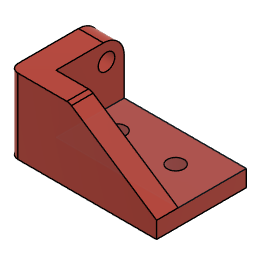
GTMS TEMPLATE (Autodesk Fusion 360 archive; units mm, degrees)
design "ROOF MOUNT"
Autodesk Fusion 360 part; units mm, degrees
(part 1 of 24)
sketch "Sketch1" plane through (0, 0, 0) normal (0, 1, 0) x (1, 0, 0)
sketch "Sketch2" plane through (0, 0, 0) normal (0, 0, 1) x (1, 0, 0)
  line L0 (0, 0) -> (7.2, 0)
  line L1 (7.2, 0) -> (7.2, 3)
  line L2 (7.2, 3) -> (14.4, 3)
  line L3 (14.4, 3) -> (14.4, 0)
  line L4 (14.4, 0) -> (17.7, 0)
  line L5 (17.7, 0) -> (17.7, 3)
  line L6 (0, 0) -> (0, 10)
  line L7 (0, 10) -> (7.2, 10)
  line L8 (7.2, 10) -> (17.7, 3)
  dimension "d1" = 7.2
  dimension "d2" = 3
  dimension "d3" = 7.2
  dimension "d4" = 3.3
  dimension "d5" = 3
  dimension "d6" = 10
  dimension "d7" = 7.2
  constraint coincident L0.start L6.start
  constraint horizontal L0
  constraint perpendicular L0 L1
  constraint perpendicular L1 L2
  constraint perpendicular L2 L3
  constraint perpendicular L3 L4
  constraint perpendicular L4 L5
  constraint perpendicular L0 L6
  constraint perpendicular L6 L7
  measures "d1" distance of L0.start L0.end
  measures "d2" distance of L0.end L1.end
  measures "d3" distance of L1.end L2.end
  measures "d4" distance of L3.end L4.end
  measures "d5" distance of L4.end L5.end
  measures "d6" distance of L0.start L6.end
  measures "d7" distance of L6.end L7.end
ref_plane "WorkPlane1" through (0, 0, 0) normal (1, 0, 0) x (0, 1, 0)
sketch "Sketch3" plane through (0, 0, 0) normal (1, 0, 0) x (0, 0, -1)
extrude "Extrude1" add sketch "Sketch2" against normal blind 2.6
sketch "Sketch4" plane through (0, 0, 0) normal (1, 0, 0) x (0, 0, -1)
  line L0 (2.6, 0) -> (10.8, 0)
  line L1 (10.8, 0) -> (10.8, 3)
  line L2 (10.8, 3) -> (2.6, 3)
  line L3 (2.6, 3) -> (2.6, 0)
  line L4 (2.6, 10) -> (8.8, 10)
  line L5 (10.8, 8) -> (10.8, 3)
  line L6 (10.8, 3) -> (2.6, 3)
  line L7 (2.6, 3) -> (2.6, 10)
  circle A0 centre (8.6724, 7.8369) radius 1
  line L8 (8.8, 10) -> (10.8, 10)
  line L9 (10.8, 10) -> (10.8, 8)
  point P0 (10.8, 10)
  dimension "d11" = 8.2
  dimension "d12" = 3
  dimension "d13" = 8.2
  dimension "d14" = 3
  dimension "d16" = 8.2
  dimension "d18" = 2
  constraint horizontal L0
  constraint perpendicular L0 L1
  constraint perpendicular L1 L2
  constraint perpendicular L2 L3
  constraint horizontal L4
  constraint perpendicular L2 L5
  constraint coincident P0 L4
  constraint coincident P0 L5
  constraint coincident P0 L8.end
  measures "d11" distance of L0.start L0.end
  measures "d12" distance of L0.end L1.end
  measures "d13" distance of L1.end L2.end
  measures "d14" distance of L2.end L0.start
  measures "d16" distance of L4.start P0
  measures "d18" diameter of A0
extrude "Extrude2" add sketch "Sketch4" along normal blind 3 contours L2 L4 L5 L6 L7 L8 L9
extrude "Extrude3" add sketch "Sketch4" along normal blind 7.2 contours L0 L1 L2 L3 L6
fillet "Fillet2" radius 1 1 edges at (7.2, 10, -1.3)
fillet "Fillet3" radius 1 1 edges at (0, 5, 0)
fillet "Fillet5" radius 1 1 edges at (16.05, 0, 0)
sketch "Sketch5" plane through (0, 0, 0) normal (0, 0, 1) x (1, 0, 0)
extrude "Extrude4" add sketch "Sketch4" along normal blind 3 contours L2 L4 L5 L6 L7 L8 L9
fillet "Fillet6" radius 2.5 1 edges at (1.5, 10, -10.8)
extrude "Extrude5" cut 1 faces at (7.2, 1, -4.4667) along direction (1, 0, 0) blind 12
extrude "Extrude6" add 1 faces at (7.2, 1, -4.4667) along direction (1, 0, 0) blind 10.5
extrude "Extrude7" cut 1 faces at (6.2333, 0, -7.2) along direction (0, 1, 0) blind 1
sketch "Sketch6" plane through (0, 3, 0) normal (0, 1, 0) x (-1, 0, 0)
  line L0 (-3, -10.8) -> (-3, -2.6)
  line L1 (-3, -2.6) -> (-17.7, -2.6)
  line L2 (-17.7, -2.6) -> (-17.7, -10.8)
  line L3 (-17.7, -10.8) -> (-3, -10.8)
sketch "Sketch7" plane through (0, 3, 0) normal (0, 1, 0) x (-1, 0, 0)
  circle A0 centre (-6, -7) radius 1
  circle A1 centre (-13, -7) radius 1
  dimension "d43" = 2
  dimension "d44" = 2
  measures "d43" diameter of A0
  measures "d44" diameter of A1
hole "Hole1" at (6, 3, -7) direction (0, -1, 0) diameter 2 depth 4 tip angle 118
hole "Hole2" at (13, 3, -7) direction (0, -1, 0) diameter 2 depth 4 tip angle 118

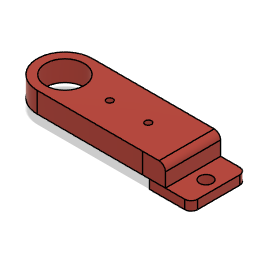
design "SERVO CAM"
Autodesk Fusion 360 part; units mm, degrees
sketch "Sketch1" plane through (0, 0, 0) normal (0, 1, 0) x (1, 0, 0)
  circle A0 centre (0, 0) radius 2.5
  line L0 (-0.0213, 4.2999) -> (16.4103, 4.3)
  line L1 (-0.0213, -4.2999) -> (16.4103, -4.3)
  arc A1 (0.0212, 4.2999) -> (0.0212, -4.2999) centre (0, 0) ccw
  arc A2 (16.3897, -4.3) -> (16.3897, 4.3) centre (16.4, 0) ccw
  point P0 (-4.3, 0)
  point P1 (25.7, 0)
  dimension "d1" = 5
  dimension "d2" = 8.6
  dimension "d12" = 16.4
  dimension "d14" = 8.6
  constraint coincident A0.centre A1.centre
  constraint concentric A0 A1
  constraint coincident L0.start A1
  constraint coincident L1.start A1
  constraint coincident L0 A1.start
  constraint coincident L1 A1.end
  constraint midpoint A1 P0
  constraint coincident L0.end A2
  constraint coincident L1.end A2
  constraint coincident L0 A2.end
  constraint coincident L1 A2.start
  measures "d1" diameter of A0
  measures "d2" diameter of A1
  measures "d12" distance of A0.centre A2.centre
  measures "d14" diameter of A2
sketch "Sketch2" plane through (0, 0, 0) normal (0, 1, 0) x (1, 0, 0)
  point P0 (-0.8314, -7.8419)
sketch "Sketch3" plane through (0, 0, 0) normal (0, 1, 0) x (1, 0, 0)
  circle A0 centre (18.5, 0) radius 1
  dimension "d16" = 2
  measures "d16" diameter of A0
extrude "Extrude2" add sketch "Sketch1" along normal blind 3.2
extrude "Extrude3" cut sketch "Sketch3" along normal blind 12
sketch "Sketch4" plane through (0, 3.2, 0) normal (0, 1, 0) x (-1, 0, 0)
  circle A0 centre (-18.5, 0) radius 1
  circle A1 centre (0, 0) radius 2.5
  arc A2 (0.0213, -4.2999) -> (0.0213, 4.2999) centre (0, 0) ccw
  line L0 (0.0213, 4.2999) -> (-16.4103, 4.3)
  arc A3 (-16.4103, 4.3) -> (-16.4103, -4.3) centre (-16.4, 0) ccw
  line L1 (-16.4103, -4.3) -> (0.0213, -4.2999)
  line L2 (-16.4103, 4.3) -> (-16.4103, -4.3)
  constraint coincident L0.end A3.start
  constraint coincident A3.end L1.start
extrude "Extrude4" cut sketch "Sketch4" against normal blind 3 contours A3 L2
extrude "Extrude5" cut 1 faces at (16.7735, 0.2, 0) along direction (0, -1, 0) blind 0.5
sketch "Sketch5" plane through (0, 0, 0) normal (0, 1, 0) x (1, 0, 0)
sketch "Sketch6" plane through (16.4103, 0, 0) normal (1, 0, 0) x (0, 0, -1)
  line L0 (4.3, 3.2) -> (-4.3, 3.2)
  line L1 (-4.3, 3.2) -> (-4.3, 0)
  line L2 (-4.3, 0) -> (4.3, 0)
  line L3 (4.3, 0) -> (4.3, 3.2)
sketch "Sketch7" plane through (0, 0, 0) normal (0, 1, 0) x (1, 0, 0)
extrude "Extrude6" add sketch "Sketch6" along normal blind 3.568
sketch "Sketch8" plane through (0, 0, 0) normal (0, 1, 0) x (1, 0, 0)
  line L0 (19.98, -4.3) -> (16.98, -4.3)
  line L1 (19.98, -4.3) -> (23.98, -4.3)
  line L2 (23.98, -4.3) -> (23.98, 7.4552)
  line L3 (20, 4.3) -> (23.98, 4.3)
  line L4 (20, 4.3) -> (17, 4.3)
  line L5 (16.98, -4.3) -> (17, 4.3)
  dimension "d33" = 3
  dimension "d34" = 4
  dimension "d35" = 3
  constraint horizontal L0
  constraint parallel L0 L1
  constraint perpendicular L1 L2
  constraint coincident L2 L3.end
  constraint perpendicular L2 L3
  constraint perpendicular L2 L4
  measures "d33" distance of L0.start L0.end
  measures "d34" distance of L0.start L1.end
  measures "d35" distance of L3.start L4.end
extrude "Extrude7" add sketch "Sketch8" against normal blind 1.4
fillet "Fillet1" radius 1 1 edges at (19.9783, 3.2, 0)
fillet "Fillet2" radius 1 1 edges at (23.98, -0.7, 4.3)
fillet "Fillet3" radius 1 1 edges at (23.98, -0.7, -4.3)
hole "Hole1" at (0, 3.2, 0) direction (0, -1, 0) diameter 6 depth 6 tip angle 180
sketch "Sketch9" plane through (0, 0, 0) normal (0, 1, 0) x (1, 0, 0)
  line L0 (0, 0) -> (26, 0)
  line L1 (20, 3) -> (24, 3)
  line L2 (24, 3) -> (22, 3)
  line L3 (22, 3) -> (22, -3)
  circle A0 centre (22, 0) radius 1
  dimension "d47" = 2
  dimension "d48" = 2
  constraint coincident L0.start origin
  constraint horizontal L0
  constraint parallel L0 L1
  constraint midpoint L1 L2.end
  constraint perpendicular L0 L3
  constraint midpoint L3 A0.centre
  measures "d47" distance of L1.end L2.end
  measures "d48" diameter of A0
hole "Hole2" at (22, 0, 0) direction (0, -1, 0) diameter 2 depth 6 tip angle 180
extrude "Extrude8" cut 1 faces at (16.9867, -0.9333, 1.4333) along direction (0.999997, 0, 0.002325) blind 0.5
delete_face "DeleteFace1" 1 faces at (17.1684, -0.9333, -4.2996)
sketch "Sketch10" plane through (0, 3.2, 0) normal (0, 1, 0) x (-1, 0, 0)
  circle A0 centre (0, 0) radius 3
  line L0 (-18.9783, 4.3) -> (-18.9783, -4.3)
  line L1 (-18.9783, -4.3) -> (-16.4103, -4.3)
  line L2 (-16.4103, -4.3) -> (0.0213, -4.2999)
  arc A1 (0.0213, -4.2999) -> (0.0213, 4.2999) centre (0, 0) ccw
  line L3 (0.0213, 4.2999) -> (-16.4103, 4.3)
  line L4 (-16.4103, 4.3) -> (-18.9783, 4.3)
  line L5 (-3, 0) -> (-4.5, 0)
  line L6 (-4.5, 0) -> (-5, 0)
  circle A2 centre (-5, 0) radius 0.5
  line L7 (-5.5, 0) -> (-6.5, 0)
  line L8 (-6.5, 0) -> (-7, 0)
  circle A3 centre (-7, 0) radius 0.5
  line L9 (-7.5, 0) -> (-8.5, 0)
  line L10 (-8.5, 0) -> (-9, 0)
  circle A4 centre (-9, 0) radius 0.5
  line L11 (-9.5, 0) -> (-10.5, 0)
  line L12 (-10.5, 0) -> (-11, 0)
  circle A5 centre (-11, 0) radius 0.5
  line L13 (-11.5, 0) -> (-12.5, 0)
  line L14 (-12.5, 0) -> (-13, 0)
  circle A6 centre (-13, 0) radius 0.5
  line L15 (-13.5, 0) -> (-14.5, 0)
  line L16 (-14.5, 0) -> (-15, 0)
  circle A7 centre (-15, 0) radius 0.5
  dimension "d54" = 1.5
  dimension "d55" = 0.5
  dimension "d56" = 1
  dimension "d57" = 1
  dimension "d58" = 0.5
  dimension "d59" = 1
  dimension "d60" = 1
  dimension "d61" = 0.5
  dimension "d62" = 1
  dimension "d63" = 1
  dimension "d64" = 0.5
  dimension "d65" = 1
  dimension "d66" = 1
  dimension "d67" = 0.5
  dimension "d68" = 1
  dimension "d69" = 1
  dimension "d70" = 0.5
  dimension "d71" = 1
  constraint coincident A0 L5.start
  constraint horizontal L5
  constraint parallel L2 L6
  constraint coincident L6.end A2.centre
  constraint coincident A2 L7.start
  constraint horizontal L7
  constraint parallel L7 L8
  constraint coincident L8.end A3.centre
  constraint coincident A3 L9.start
  constraint horizontal L9
  constraint parallel L9 L10
  constraint coincident L10.end A4.centre
  constraint coincident A4 L11.start
  constraint horizontal L11
  constraint parallel L11 L12
  constraint coincident L12.end A5.centre
  constraint coincident A5 L13.start
  constraint parallel L2 L13
  constraint horizontal L14
  constraint coincident L14.end A6.centre
  constraint coincident A6 L15.start
  constraint parallel L2 L15
  constraint parallel L15 L16
  constraint coincident L16.end A7.centre
  measures "d54" distance of L5.start L5.end
  measures "d55" distance of L5.end L6.end
  measures "d56" diameter of A2
  measures "d57" distance of L7.start L7.end
  measures "d58" distance of L7.end L8.end
  measures "d59" diameter of A3
  measures "d60" distance of L9.start L9.end
  measures "d61" distance of L9.end L10.end
  measures "d62" diameter of A4
  measures "d63" distance of L11.start L11.end
  measures "d64" distance of L11.end L12.end
  measures "d65" diameter of A5
  measures "d66" distance of L13.start L13.end
  measures "d67" distance of L13.end L14.end
  measures "d68" diameter of A6
  measures "d69" distance of L15.start L15.end
  measures "d70" distance of L15.end L16.end
  measures "d71" diameter of A7
hole "Hole3" at (7, 3.2, 0) direction (0, -1, 0) diameter 1 depth 10 tip angle 118
hole "Hole4" at (13, 3.2, 0) direction (0, -1, 0) diameter 1 depth 10 tip angle 118
extrude "Extrude1" [suppressed]

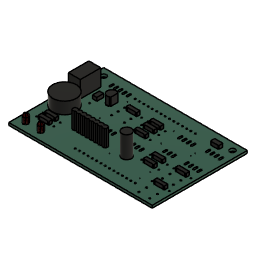
design "IO Daughter Board"
Autodesk Fusion 360 part; units mm, degrees
sketch "Outline" plane through (0, 0, 0) normal (0, 0, 1) x (1, 0, 0)
  line L0 (0, 0) -> (0, 56.3)
  arc A0 (0, 56.3381) -> (0, 56.2619) centre (0, 56.3) ccw
  line L1 (85, 56.3) -> (85, 0)
  arc A1 (85.0381, 56.3) -> (84.9619, 56.3) centre (85, 56.3) ccw
  arc A2 (0.0381, 56.3) -> (-0.0381, 56.3) centre (0, 56.3) ccw
  arc A3 (-0.0381, 0) -> (0.0381, 0) centre (0, 0) ccw
  line L2 (0, 56.3) -> (85, 56.3)
  arc A4 (0, 0.0381) -> (0, -0.0381) centre (0, 0) ccw
  arc A5 (85, 56.2619) -> (85, 56.3381) centre (85, 56.3) ccw
  arc A6 (85, -0.0381) -> (85, 0.0381) centre (85, 0) ccw
  line L3 (85, 0) -> (0, 0)
  arc A7 (84.9619, 0) -> (85.0381, 0) centre (85, 0) ccw
sketch "Top SIlkscreen" plane through (0, 0, 0) normal (0, 0, 1) x (1, 0, 0)
  line L0 (55.2958, 9.3303) -> (56.4642, 9.7197)
  arc A0 (55.2878, 9.3544) -> (55.3038, 9.3062) centre (55.2958, 9.3303) ccw
  arc A1 (52.7304, 13.311) -> (52.7812, 13.311) centre (52.7558, 13.311) ccw
  line L1 (56.1721, 9.6224) -> (56.1721, 9.0382)
  arc A2 (56.4722, 9.6956) -> (56.4562, 9.7438) centre (56.4642, 9.7197) ccw
  arc A3 (53.6646, 12.8425) -> (53.6646, 12.7917) centre (53.6646, 12.8171) ccw
  arc A4 (53.9242, 13.2856) -> (53.9242, 13.3364) centre (53.9242, 13.311) ccw
  arc A5 (53.9242, 10.5777) -> (53.9242, 10.6285) centre (53.9242, 10.6031) ccw
  arc A6 (53.6392, 10.1487) -> (53.69, 10.1487) centre (53.6646, 10.1487) ccw
  arc A7 (52.6347, 11.7855) -> (52.6173, 11.7377) centre (52.626, 11.7616) ccw
  arc A8 (53.8988, 12.5575) -> (53.9496, 12.5575) centre (53.9242, 12.5575) ccw
  arc A9 (52.7304, 12.4601) -> (52.7812, 12.4601) centre (52.7558, 12.4601) ccw
  line L2 (53.4049, 10.6031) -> (53.9242, 10.6031)
  arc A10 (53.7619, 12.168) -> (53.9242, 12.5575) centre (53.3757, 12.5575) ccw
  arc A11 (53.8988, 13.6356) -> (53.9496, 13.6356) centre (53.9242, 13.6356) ccw
  arc A12 (52.7638, 14.8408) -> (52.7478, 14.7926) centre (52.7558, 14.8167) ccw
  line L3 (53.9242, 13.6356) -> (53.9242, 13.311)
  arc A13 (52.8532, 12.7522) -> (52.7558, 12.4601) centre (53.2426, 12.4601) ccw
  arc A14 (53.0154, 12.1751) -> (53.0154, 12.2259) centre (53.0154, 12.2005) ccw
  arc A15 (53.6646, 12.8171) -> (53.4374, 12.6873) centre (53.6646, 12.5534) ccw
  line L4 (52.7558, 14.8167) -> (53.9242, 15.2061)
  arc A16 (53.9162, 14.4031) -> (53.9322, 14.4513) centre (53.9242, 14.4272) ccw
  arc A17 (53.69, 10.7978) -> (53.6392, 10.7978) centre (53.6646, 10.7978) ccw
  arc A18 (54.0453, 11.2184) -> (54.0627, 11.2662) centre (54.054, 11.2423) ccw
  arc A19 (53.0804, 13.9347) -> (53.0804, 13.9855) centre (53.0804, 13.9601) ccw
  arc A20 (53.8988, 13.311) -> (53.9496, 13.311) centre (53.9242, 13.311) ccw
  line L5 (56.4642, 8.9408) -> (55.2958, 9.3303)
  arc A21 (52.7812, 13.6356) -> (52.7304, 13.6356) centre (52.7558, 13.6356) ccw
  line L6 (53.9242, 14.4272) -> (52.7558, 14.8167)
  line L7 (53.6321, 15.1088) -> (53.6321, 14.5246)
  arc A22 (52.8735, 12.737) -> (52.8328, 12.7674) centre (52.8531, 12.7522) ccw
  arc A23 (53.0804, 13.9855) -> (53.0804, 13.9347) centre (53.0804, 13.9601) ccw
  arc A24 (55.3038, 9.3544) -> (55.2878, 9.3062) centre (55.2958, 9.3303) ccw
  arc A25 (53.744, 12.186) -> (53.7798, 12.15) centre (53.7619, 12.168) ccw
  arc A26 (53.0154, 12.2005) -> (53.2426, 12.3303) centre (53.0154, 12.4642) ccw
  arc A27 (52.7628, 10.4328) -> (52.7488, 10.3839) centre (52.7558, 10.4084) ccw
  arc A28 (52.7558, 12.4601) -> (53.0154, 12.2005) centre (53.0154, 12.4601) ccw
  line L8 (53.9242, 13.311) -> (52.7558, 13.311)
  arc A29 (53.2203, 12.3424) -> (53.2649, 12.3181) centre (53.2426, 12.3302) ccw
  arc A30 (52.7812, 12.4601) -> (52.7304, 12.4601) centre (52.7558, 12.4601) ccw
  arc A31 (53.4049, 10.6285) -> (53.4049, 10.5777) centre (53.4049, 10.6031) ccw
  arc A32 (53.0154, 12.2259) -> (53.0154, 12.1751) centre (53.0154, 12.2005) ccw
  arc A33 (52.7304, 13.6356) -> (52.7812, 13.6356) centre (52.7558, 13.6356) ccw
  line L9 (53.0804, 13.9601) -> (53.5996, 13.9601)
  arc A34 (53.9496, 12.5575) -> (53.8988, 12.5575) centre (53.9242, 12.5575) ccw
  arc A35 (53.5996, 13.9855) -> (53.5996, 13.9347) centre (53.5996, 13.9601) ccw
  arc A36 (53.5996, 13.9347) -> (53.5996, 13.9855) centre (53.5996, 13.9601) ccw
  line L10 (53.4374, 12.6873) -> (53.2426, 12.3303)
  arc A37 (53.0804, 13.9601) -> (52.7558, 13.6356) centre (53.0804, 13.6355) ccw
  arc A38 (53.9242, 13.6356) -> (53.5996, 13.9601) centre (53.5996, 13.6355) ccw
  arc A39 (53.9242, 12.5575) -> (53.6646, 12.8171) centre (53.6646, 12.5575) ccw
  arc A40 (53.2645, 12.3174) -> (53.2208, 12.3432) centre (53.2427, 12.3303) ccw
  arc A41 (53.4155, 12.7002) -> (53.4593, 12.6744) centre (53.4374, 12.6873) ccw
  arc A42 (53.4597, 12.6751) -> (53.4151, 12.6995) centre (53.4374, 12.6873) ccw
  arc A43 (53.9322, 15.182) -> (53.9162, 15.2302) centre (53.9242, 15.2061) ccw
  arc A44 (56.4562, 8.9167) -> (56.4722, 8.9649) centre (56.4642, 8.9408) ccw
  arc A45 (53.6646, 12.7917) -> (53.6646, 12.8425) centre (53.6646, 12.8171) ccw
  arc A46 (52.7478, 14.8408) -> (52.7638, 14.7926) centre (52.7558, 14.8167) ccw
  line L11 (54.054, 11.2423) -> (52.626, 11.7616)
  arc A47 (53.6575, 15.1088) -> (53.6067, 15.1088) centre (53.6321, 15.1088) ccw
  line L12 (52.7558, 13.311) -> (52.7558, 13.6356)
  arc A48 (52.7558, 13.3364) -> (52.7558, 13.2856) centre (52.7558, 13.311) ccw
  arc A49 (53.6067, 14.5246) -> (53.6575, 14.5246) centre (53.6321, 14.5246) ccw
  arc A50 (53.9496, 13.6356) -> (53.8988, 13.6356) centre (53.9242, 13.6356) ccw
  arc A51 (55.3212, 12.4601) -> (55.2704, 12.4601) centre (55.2958, 12.4601) ccw
  arc A52 (56.4642, 10.5382) -> (56.2046, 10.7978) centre (56.2046, 10.5382) ccw
  arc A53 (56.2046, 10.7724) -> (56.2046, 10.8232) centre (56.2046, 10.7978) ccw
  arc A54 (41.0619, 54.9233) -> (41.2242, 55.1504) centre (40.9841, 55.1504) ccw
  arc A55 (56.2046, 12.8425) -> (56.2046, 12.7917) centre (56.2046, 12.8171) ccw
  arc A56 (41.0537, 54.9473) -> (41.0702, 54.8992) centre (41.062, 54.9233) ccw
  line L13 (56.4642, 10.1487) -> (56.4642, 10.5382)
  arc A57 (56.4388, 12.5575) -> (56.4896, 12.5575) centre (56.4642, 12.5575) ccw
  arc A58 (41.1988, 55.1504) -> (41.2496, 55.1504) centre (41.2242, 55.1504) ccw
  arc A59 (55.2958, 10.1741) -> (55.2958, 10.1233) centre (55.2958, 10.1487) ccw
  arc A60 (40.64, 54.8513) -> (40.64, 54.8005) centre (40.64, 54.8259) ccw
  arc A61 (56.0747, 10.7724) -> (56.0747, 10.8232) centre (56.0747, 10.7978) ccw
  arc A62 (41.2242, 55.1504) -> (41.0619, 55.3776) centre (40.984, 55.1504) ccw
  arc A63 (41.0508, 55.3548) -> (41.0731, 55.4005) centre (41.0619, 55.3777) ccw
  arc A64 (55.7897, 10.1487) -> (55.8405, 10.1487) centre (55.8151, 10.1487) ccw
  arc A65 (55.3212, 10.7978) -> (55.2704, 10.7978) centre (55.2958, 10.7978) ccw
  arc A66 (56.4388, 10.1487) -> (56.4896, 10.1487) centre (56.4642, 10.1487) ccw
  line L14 (55.2958, 10.1487) -> (55.2958, 10.7978)
  arc A67 (56.4642, 12.5575) -> (56.2046, 12.8171) centre (56.2046, 12.5575) ccw
  arc A68 (34.8822, 28.7456) -> (34.8662, 28.7938) centre (34.8742, 28.7697) ccw
  arc A69 (40.64, 55.5004) -> (40.64, 55.4496) centre (40.64, 55.475) ccw
  arc A70 (56.4896, 10.5382) -> (56.4388, 10.5382) centre (56.4642, 10.5382) ccw
  arc A71 (56.3019, 12.168) -> (56.4642, 12.5575) centre (55.9157, 12.5575) ccw
  arc A72 (55.1747, 11.7855) -> (55.1573, 11.7377) centre (55.166, 11.7616) ccw
  arc A73 (55.5554, 12.1751) -> (55.5554, 12.2259) centre (55.5554, 12.2005) ccw
  arc A74 (56.2046, 10.8232) -> (56.2046, 10.7724) centre (56.2046, 10.7978) ccw
  arc A75 (55.8405, 10.5382) -> (55.7897, 10.5382) centre (55.8151, 10.5382) ccw
  arc A76 (41.0702, 55.4017) -> (41.0537, 55.3536) centre (41.0619, 55.3777) ccw
  arc A77 (55.8151, 10.1233) -> (55.8151, 10.1741) centre (55.8151, 10.1487) ccw
  line L15 (56.594, 11.2423) -> (55.166, 11.7616)
  line L16 (55.8151, 10.5382) -> (55.8151, 10.1487)
  arc A78 (40.9487, 54.871) -> (40.9804, 54.9106) centre (40.9646, 54.8908) ccw
  line L17 (40.9646, 54.8908) -> (40.3154, 55.4101)
  arc A79 (41.0619, 55.3776) -> (40.64, 55.475) centre (40.6399, 54.5123) ccw
  arc A80 (40.3313, 55.4299) -> (40.2996, 55.3903) centre (40.3154, 55.4101) ccw
  line L18 (43.7642, 52.5018) -> (42.5958, 52.5018)
  line L19 (42.5958, 52.5018) -> (42.5958, 52.8264)
  arc A81 (56.0747, 10.8232) -> (56.0747, 10.7724) centre (56.0747, 10.7978) ccw
  arc A82 (55.2704, 10.1487) -> (55.3212, 10.1487) centre (55.2958, 10.1487) ccw
  line L20 (56.2046, 10.7978) -> (56.0747, 10.7978)
  arc A83 (56.1975, 9.6224) -> (56.1467, 9.6224) centre (56.1721, 9.6224) ccw
  arc A84 (56.0747, 10.7978) -> (55.8151, 10.5382) centre (56.0747, 10.5382) ccw
  line L21 (55.8151, 10.1487) -> (55.2958, 10.1487)
  arc A85 (55.2958, 12.4601) -> (55.5554, 12.2005) centre (55.5554, 12.4601) ccw
  arc A86 (55.3932, 12.7522) -> (55.2958, 12.4601) centre (55.7826, 12.4601) ccw
  arc A87 (56.284, 12.186) -> (56.3198, 12.15) centre (56.3019, 12.168) ccw
  line L22 (26.6051, 29.6644) -> (26.6051, 29.2749)
  arc A88 (56.4896, 12.5575) -> (56.4388, 12.5575) centre (56.4642, 12.5575) ccw
  arc A89 (40.64, 55.4496) -> (40.64, 55.5004) centre (40.64, 55.475) ccw
  arc A90 (40.2069, 55.4005) -> (40.2292, 55.3548) centre (40.218, 55.3777) ccw
  arc A91 (41.0731, 54.9004) -> (41.0508, 54.9461) centre (41.062, 54.9233) ccw
  arc A92 (56.4388, 10.5382) -> (56.4896, 10.5382) centre (56.4642, 10.5382) ccw
  line L23 (43.9972, 30.4165) -> (44.6322, 30.4165)
  arc A93 (40.0304, 55.1504) -> (40.0812, 55.1504) centre (40.0558, 55.1504) ccw
  arc A94 (41.2496, 55.1504) -> (41.1988, 55.1504) centre (41.2242, 55.1504) ccw
  line L24 (29.1451, 28.4452) -> (29.1451, 28.6399)
  arc A95 (56.5853, 11.2184) -> (56.6027, 11.2662) centre (56.594, 11.2423) ccw
  arc A96 (47.9679, 10.7724) -> (47.9679, 10.8232) centre (47.9679, 10.7978) ccw
  line L25 (26.6051, 29.2749) -> (26.0858, 29.2749)
  arc A97 (40.64, 55.475) -> (40.2181, 55.3776) centre (40.6401, 54.5123) ccw
  arc A98 (56.1467, 9.0382) -> (56.1975, 9.0382) centre (56.1721, 9.0382) ccw
  arc A99 (40.64, 54.8259) -> (41.0619, 54.9233) centre (40.6399, 55.7886) ccw
  arc A100 (55.7897, 10.5382) -> (55.8405, 10.5382) centre (55.8151, 10.5382) ccw
  arc A101 (45.8526, 54.3066) -> (45.8526, 54.3574) centre (45.8526, 54.332) ccw
  arc A102 (42.9204, 53.1509) -> (42.5958, 52.8264) centre (42.9204, 52.8263) ccw
  line L26 (43.7642, 52.8264) -> (43.7642, 52.5018)
  arc A103 (45.8526, 53.7083) -> (45.8526, 53.6575) centre (45.8526, 53.6829) ccw
  arc A104 (45.8526, 53.1763) -> (45.8526, 53.1255) centre (45.8526, 53.1509) ccw
  arc A105 (45.8526, 54.3574) -> (45.8526, 54.3066) centre (45.8526, 54.332) ccw
  arc A106 (45.2684, 53.7478) -> (45.2684, 54.2671) centre (45.2684, 54.0075) ccw
  arc A107 (43.7388, 52.8264) -> (43.7896, 52.8264) centre (43.7642, 52.8264) ccw
  arc A108 (45.3334, 53.1255) -> (45.3334, 53.1763) centre (45.3334, 53.1509) ccw
  arc A109 (44.9834, 52.5018) -> (45.0342, 52.5018) centre (45.0088, 52.5018) ccw
  arc A110 (45.2684, 54.2925) -> (45.2684, 54.2417) centre (45.2684, 54.2671) ccw
  arc A111 (45.2684, 53.7732) -> (45.2684, 53.7224) centre (45.2684, 53.7478) ccw
  arc A112 (42.9853, 53.6829) -> (43.2449, 53.9425) centre (42.9853, 53.9425) ccw
  arc A113 (42.9204, 53.6575) -> (42.9204, 53.7083) centre (42.9204, 53.6829) ccw
  arc A114 (42.9204, 54.3066) -> (42.9204, 54.3574) centre (42.9204, 54.332) ccw
  arc A115 (43.2449, 54.3066) -> (43.2449, 54.3574) centre (43.2449, 54.332) ccw
  arc A116 (43.2449, 54.3574) -> (43.2449, 54.3066) centre (43.2449, 54.332) ccw
  arc A117 (42.9204, 53.7083) -> (42.9204, 53.6575) centre (42.9204, 53.6829) ccw
  arc A118 (42.9853, 53.6575) -> (42.9853, 53.7083) centre (42.9853, 53.6829) ccw
  arc A119 (42.9204, 53.1763) -> (42.9204, 53.1255) centre (42.9204, 53.1509) ccw
  arc A120 (43.2703, 53.9425) -> (43.2195, 53.9425) centre (43.2449, 53.9425) ccw
  arc A121 (42.5704, 52.8264) -> (42.6212, 52.8264) centre (42.5958, 52.8264) ccw
  arc A122 (43.2703, 54.332) -> (43.2195, 54.332) centre (43.2449, 54.332) ccw
  line L27 (42.9853, 53.6829) -> (42.9204, 53.6829)
  line L28 (42.9204, 54.332) -> (43.2449, 54.332)
  arc A123 (43.7642, 53.8127) -> (43.2449, 54.332) centre (43.2449, 53.8127) ccw
  arc A124 (46.1772, 52.4764) -> (46.1772, 52.5272) centre (46.1772, 52.5018) ccw
  arc A125 (45.0342, 52.8264) -> (44.9834, 52.8264) centre (45.0088, 52.8264) ccw
  line L29 (42.9204, 53.1509) -> (43.4396, 53.1509)
  arc A126 (45.0088, 52.5272) -> (45.0088, 52.4764) centre (45.0088, 52.5018) ccw
  line L30 (45.0088, 52.5018) -> (45.0088, 52.8264)
  line L31 (45.3334, 53.1509) -> (45.8526, 53.1509)
  arc A127 (42.9204, 54.332) -> (42.9204, 53.6829) centre (42.9204, 54.0074) ccw
  arc A128 (43.7388, 52.5018) -> (43.7896, 52.5018) centre (43.7642, 52.5018) ccw
  arc A129 (45.3334, 53.1763) -> (45.3334, 53.1255) centre (45.3334, 53.1509) ccw
  arc A130 (46.1518, 52.8264) -> (46.2026, 52.8264) centre (46.1772, 52.8264) ccw
  arc A131 (43.7642, 52.8264) -> (43.4396, 53.1509) centre (43.4396, 52.8263) ccw
  line L32 (46.1772, 52.8264) -> (46.1772, 52.5018)
  arc A132 (45.3334, 53.1509) -> (45.0088, 52.8264) centre (45.3334, 52.8263) ccw
  arc A133 (45.8526, 53.6575) -> (45.8526, 53.7083) centre (45.8526, 53.6829) ccw
  arc A134 (43.7896, 52.8264) -> (43.7388, 52.8264) centre (43.7642, 52.8264) ccw
  arc A135 (46.1772, 52.8264) -> (45.8526, 53.1509) centre (45.8526, 52.8263) ccw
  arc A136 (42.9853, 53.7083) -> (42.9853, 53.6575) centre (42.9853, 53.6829) ccw
  arc A137 (45.2684, 54.2417) -> (45.2684, 54.2925) centre (45.2684, 54.2671) ccw
  arc A138 (45.2684, 53.7224) -> (45.2684, 53.7732) centre (45.2684, 53.7478) ccw
  arc A139 (42.5704, 52.5018) -> (42.6212, 52.5018) centre (42.5958, 52.5018) ccw
  arc A140 (43.4396, 53.1255) -> (43.4396, 53.1763) centre (43.4396, 53.1509) ccw
  arc A141 (43.2195, 53.9425) -> (43.2703, 53.9425) centre (43.2449, 53.9425) ccw
  line L33 (46.1772, 52.5018) -> (45.0088, 52.5018)
  arc A142 (45.8526, 53.1255) -> (45.8526, 53.1763) centre (45.8526, 53.1509) ccw
  arc A143 (42.5958, 52.5272) -> (42.5958, 52.4764) centre (42.5958, 52.5018) ccw
  arc A144 (42.9204, 53.1255) -> (42.9204, 53.1763) centre (42.9204, 53.1509) ccw
  arc A145 (42.9204, 54.3574) -> (42.9204, 54.3066) centre (42.9204, 54.332) ccw
  arc A146 (46.1518, 52.5018) -> (46.2026, 52.5018) centre (46.1772, 52.5018) ccw
  arc A147 (42.6212, 52.8264) -> (42.5704, 52.8264) centre (42.5958, 52.8264) ccw
  arc A148 (43.7388, 53.8127) -> (43.7896, 53.8127) centre (43.7642, 53.8127) ccw
  arc A149 (43.4396, 53.1763) -> (43.4396, 53.1255) centre (43.4396, 53.1509) ccw
  line L34 (43.2449, 54.332) -> (43.2449, 53.9425)
  arc A150 (44.9834, 52.8264) -> (45.0342, 52.8264) centre (45.0088, 52.8264) ccw
  arc A151 (43.7642, 52.4764) -> (43.7642, 52.5272) centre (43.7642, 52.5018) ccw
  arc A152 (45.8526, 53.6829) -> (45.8526, 54.332) centre (45.8526, 54.0074) ccw
  arc A153 (46.2026, 52.8264) -> (46.1518, 52.8264) centre (46.1772, 52.8264) ccw
  arc A154 (45.8526, 54.332) -> (45.8526, 53.6829) centre (45.8526, 54.0074) ccw
  arc A155 (45.2684, 54.2671) -> (45.2684, 53.7478) centre (45.2684, 54.0075) ccw
  arc A156 (51.0596, 54.3066) -> (51.0596, 54.3574) centre (51.0596, 54.332) ccw
  arc A157 (48.0004, 53.189) -> (48.0004, 53.2398) centre (48.0004, 53.2144) ccw
  line L35 (47.6758, 53.7464) -> (47.6758, 54.3955)
  arc A158 (50.5404, 53.1509) -> (50.2158, 52.8264) centre (50.5404, 52.8263) ccw
  arc A159 (47.6758, 52.5907) -> (47.6758, 52.5399) centre (47.6758, 52.5653) ccw
  arc A160 (50.2412, 54.2022) -> (50.1904, 54.2022) centre (50.2158, 54.2022) ccw
  arc A161 (51.0596, 53.6575) -> (51.0596, 53.7083) centre (51.0596, 53.6829) ccw
  arc A162 (47.6504, 53.7464) -> (47.7012, 53.7464) centre (47.6758, 53.7464) ccw
  line L36 (53.9242, 52.5018) -> (52.7558, 52.5018)
  arc A163 (47.7012, 52.8899) -> (47.6504, 52.8899) centre (47.6758, 52.8899) ccw
  arc A164 (47.6504, 52.5653) -> (47.7012, 52.5653) centre (47.6758, 52.5653) ccw
  arc A165 (48.5196, 53.189) -> (48.5196, 53.2398) centre (48.5196, 53.2144) ccw
  arc A166 (48.8188, 52.8899) -> (48.8696, 52.8899) centre (48.8442, 52.8899) ccw
  arc A167 (50.5404, 53.1763) -> (50.5404, 53.1255) centre (50.5404, 53.1509) ccw
  arc A168 (48.0004, 53.2144) -> (47.6758, 52.8899) centre (48.0004, 52.8898) ccw
  line L37 (51.3842, 52.8264) -> (51.3842, 52.5018)
  arc A169 (51.0596, 53.1763) -> (51.0596, 53.1255) centre (51.0596, 53.1509) ccw
  arc A170 (51.3588, 52.5018) -> (51.4096, 52.5018) centre (51.3842, 52.5018) ccw
  arc A171 (51.3842, 52.8264) -> (51.0596, 53.1509) centre (51.0596, 52.8263) ccw
  arc A172 (47.6826, 54.42) -> (47.669, 54.371) centre (47.6758, 54.3955) ccw
  arc A173 (50.1904, 52.8264) -> (50.2412, 52.8264) centre (50.2158, 52.8264) ccw
  line L38 (47.6758, 54.3955) -> (48.8442, 54.071)
  line L39 (50.5404, 53.1509) -> (51.0596, 53.1509)
  arc A174 (51.0596, 53.1255) -> (51.0596, 53.1763) centre (51.0596, 53.1509) ccw
  arc A175 (51.4096, 52.8264) -> (51.3588, 52.8264) centre (51.3842, 52.8264) ccw
  line L40 (48.8442, 52.8899) -> (48.8442, 52.5653)
  arc A176 (50.9947, 54.332) -> (50.7351, 54.0724) centre (50.9947, 54.0724) ccw
  arc A177 (50.7605, 54.0724) -> (50.7097, 54.0724) centre (50.7351, 54.0724) ccw
  arc A178 (47.7012, 54.3955) -> (47.6504, 54.3955) centre (47.6758, 54.3955) ccw
  arc A179 (50.9947, 54.3066) -> (50.9947, 54.3574) centre (50.9947, 54.332) ccw
  line L41 (50.9947, 54.332) -> (51.0596, 54.332)
  arc A180 (51.0596, 53.6829) -> (51.0596, 54.332) centre (51.0596, 54.0074) ccw
  arc A181 (47.6504, 52.8899) -> (47.7012, 52.8899) centre (47.6758, 52.8899) ccw
  line L42 (48.0004, 53.2144) -> (48.5196, 53.2144)
  arc A182 (48.5196, 53.2398) -> (48.5196, 53.189) centre (48.5196, 53.2144) ccw
  arc A183 (51.3842, 52.4764) -> (51.3842, 52.5272) centre (51.3842, 52.5018) ccw
  arc A184 (48.8374, 54.0465) -> (48.851, 54.0954) centre (48.8442, 54.0709) ccw
  arc A185 (51.3588, 52.8264) -> (51.4096, 52.8264) centre (51.3842, 52.8264) ccw
  arc A186 (48.8442, 52.8899) -> (48.5196, 53.2144) centre (48.5196, 52.8898) ccw
  arc A187 (51.0596, 54.3574) -> (51.0596, 54.3066) centre (51.0596, 54.332) ccw
  line L43 (50.2158, 52.5018) -> (50.2158, 52.8264)
  arc A188 (50.7351, 53.7083) -> (50.7351, 53.6575) centre (50.7351, 53.6829) ccw
  arc A189 (50.5404, 53.1255) -> (50.5404, 53.1763) centre (50.5404, 53.1509) ccw
  arc A190 (50.7351, 53.6575) -> (50.7351, 53.7083) centre (50.7351, 53.6829) ccw
  arc A191 (50.2158, 54.2022) -> (50.7351, 53.6829) centre (50.7351, 54.2022) ccw
  arc A192 (47.6758, 53.7718) -> (47.6758, 53.721) centre (47.6758, 53.7464) ccw
  arc A193 (50.2158, 52.5272) -> (50.2158, 52.4764) centre (50.2158, 52.5018) ccw
  arc A194 (50.1904, 52.5018) -> (50.2412, 52.5018) centre (50.2158, 52.5018) ccw
  arc A195 (50.7097, 54.0724) -> (50.7605, 54.0724) centre (50.7351, 54.0724) ccw
  arc A196 (50.9947, 54.3574) -> (50.9947, 54.3066) centre (50.9947, 54.332) ccw
  line L44 (47.6758, 52.5653) -> (47.6758, 52.8899)
  arc A197 (48.8696, 52.8899) -> (48.8188, 52.8899) centre (48.8442, 52.8899) ccw
  arc A198 (48.8442, 52.5399) -> (48.8442, 52.5907) centre (48.8442, 52.5653) ccw
  arc A199 (47.8056, 53.721) -> (47.8056, 53.7718) centre (47.8056, 53.7464) ccw
  line L45 (47.8056, 53.7464) -> (47.6758, 53.7464)
  arc A200 (48.0004, 53.2398) -> (48.0004, 53.189) centre (48.0004, 53.2144) ccw
  line L46 (51.3842, 52.5018) -> (50.2158, 52.5018)
  line L47 (48.8442, 52.5653) -> (47.6758, 52.5653)
  arc A201 (50.2412, 52.8264) -> (50.1904, 52.8264) centre (50.2158, 52.8264) ccw
  arc A202 (48.8188, 52.5653) -> (48.8696, 52.5653) centre (48.8442, 52.5653) ccw
  arc A203 (50.7097, 53.6829) -> (50.7605, 53.6829) centre (50.7351, 53.6829) ccw
  line L48 (50.7351, 53.6829) -> (50.7351, 54.0724)
  arc A204 (51.0596, 53.7083) -> (51.0596, 53.6575) centre (51.0596, 53.6829) ccw
  line L49 (51.0596, 53.6829) -> (50.7351, 53.6829)
  line L50 (56.4642, 52.5018) -> (55.2958, 52.5018)
  arc A205 (40.2263, 55.3536) -> (40.2098, 55.4017) centre (40.2181, 55.3776) ccw
  arc A206 (53.5996, 53.1255) -> (53.5996, 53.1763) centre (53.5996, 53.1509) ccw
  arc A207 (53.9496, 52.8264) -> (53.8988, 52.8264) centre (53.9242, 52.8264) ccw
  arc A208 (54.6885, 2.4638) -> (54.6885, 2.5146) centre (54.6885, 2.4892) ccw
  arc A209 (55.2704, 52.5018) -> (55.3212, 52.5018) centre (55.2958, 52.5018) ccw
  arc A210 (55.6204, 53.1255) -> (55.6204, 53.1763) centre (55.6204, 53.1509) ccw
  arc A211 (53.0804, 53.1509) -> (52.7558, 52.8264) centre (53.0804, 52.8263) ccw
  arc A212 (56.4388, 52.8264) -> (56.4896, 52.8264) centre (56.4642, 52.8264) ccw
  line L51 (52.7558, 52.5018) -> (52.7558, 52.8264)
  arc A213 (53.9242, 52.4764) -> (53.9242, 52.5272) centre (53.9242, 52.5018) ccw
  line L52 (26.0858, 30.353) -> (27.2542, 30.7425)
  arc A214 (54.4542, 1.5804) -> (54.4034, 1.5804) centre (54.4288, 1.5804) ccw
  line L53 (53.6646, 54.332) -> (53.5347, 54.332)
  arc A215 (26.8647, 29.8986) -> (26.8647, 29.9494) centre (26.8647, 29.924) ccw
  arc A216 (53.6646, 54.3066) -> (53.6646, 54.3574) centre (53.6646, 54.332) ccw
  arc A217 (53.5347, 54.3574) -> (53.5347, 54.3066) centre (53.5347, 54.332) ccw
  arc A218 (53.5347, 54.332) -> (53.2751, 54.0724) centre (53.5347, 54.0724) ccw
  arc A219 (53.5347, 54.3066) -> (53.5347, 54.3574) centre (53.5347, 54.332) ccw
  arc A220 (53.5996, 53.1763) -> (53.5996, 53.1255) centre (53.5996, 53.1509) ccw
  arc A221 (53.8988, 54.0724) -> (53.9496, 54.0724) centre (53.9242, 54.0724) ccw
  arc A222 (52.7304, 52.8264) -> (52.7812, 52.8264) centre (52.7558, 52.8264) ccw
  arc A223 (53.9242, 54.0724) -> (53.6646, 54.332) centre (53.6646, 54.0724) ccw
  arc A224 (53.8988, 53.6829) -> (53.9496, 53.6829) centre (53.9242, 53.6829) ccw
  arc A225 (52.7558, 53.7083) -> (52.7558, 53.6575) centre (52.7558, 53.6829) ccw
  arc A226 (34.8662, 27.9667) -> (34.8822, 28.0149) centre (34.8742, 27.9908) ccw
  arc A227 (53.2497, 53.6829) -> (53.3005, 53.6829) centre (53.2751, 53.6829) ccw
  arc A228 (53.3005, 54.0724) -> (53.2497, 54.0724) centre (53.2751, 54.0724) ccw
  arc A229 (53.0804, 53.1255) -> (53.0804, 53.1763) centre (53.0804, 53.1509) ccw
  arc A230 (53.2751, 53.6575) -> (53.2751, 53.7083) centre (53.2751, 53.6829) ccw
  arc A231 (52.7812, 54.332) -> (52.7304, 54.332) centre (52.7558, 54.332) ccw
  arc A232 (56.4642, 52.4764) -> (56.4642, 52.5272) centre (56.4642, 52.5018) ccw
  arc A233 (51.1246, 29.8986) -> (51.1246, 29.9494) centre (51.1246, 29.924) ccw
  line L54 (29.7942, 28.6399) -> (29.7942, 28.2504)
  arc A234 (52.7812, 52.8264) -> (52.7304, 52.8264) centre (52.7558, 52.8264) ccw
  arc A235 (53.8988, 52.5018) -> (53.9496, 52.5018) centre (53.9242, 52.5018) ccw
  line L55 (53.9242, 52.8264) -> (53.9242, 52.5018)
  arc A236 (53.2497, 54.0724) -> (53.3005, 54.0724) centre (53.2751, 54.0724) ccw
  arc A237 (54.9481, 2.4638) -> (54.9481, 2.5146) centre (54.9481, 2.4892) ccw
  arc A238 (55.3212, 52.8264) -> (55.2704, 52.8264) centre (55.2958, 52.8264) ccw
  arc A239 (53.0804, 53.1763) -> (53.0804, 53.1255) centre (53.0804, 53.1509) ccw
  arc A240 (55.2958, 52.5272) -> (55.2958, 52.4764) centre (55.2958, 52.5018) ccw
  arc A241 (53.6646, 54.3574) -> (53.6646, 54.3066) centre (53.6646, 54.332) ccw
  arc A242 (55.6204, 53.1509) -> (55.2958, 52.8264) centre (55.6204, 52.8263) ccw
  arc A243 (55.2704, 52.8264) -> (55.3212, 52.8264) centre (55.2958, 52.8264) ccw
  arc A244 (52.7304, 52.5018) -> (52.7812, 52.5018) centre (52.7558, 52.5018) ccw
  arc A245 (53.8988, 52.8264) -> (53.9496, 52.8264) centre (53.9242, 52.8264) ccw
  arc A246 (53.9496, 54.0724) -> (53.8988, 54.0724) centre (53.9242, 54.0724) ccw
  line L56 (52.7558, 53.6829) -> (52.7558, 54.332)
  arc A247 (52.7304, 53.6829) -> (52.7812, 53.6829) centre (52.7558, 53.6829) ccw
  arc A248 (52.7558, 52.5272) -> (52.7558, 52.4764) centre (52.7558, 52.5018) ccw
  arc A249 (28.8854, 28.0162) -> (28.8854, 27.9654) centre (28.8854, 27.9908) ccw
  arc A250 (26.0778, 30.3771) -> (26.0938, 30.3289) centre (26.0858, 30.353) ccw
  line L57 (53.0804, 53.1509) -> (53.5996, 53.1509)
  arc A251 (26.0604, 29.2749) -> (26.1112, 29.2749) centre (26.0858, 29.2749) ccw
  arc A252 (33.7138, 28.4044) -> (33.6978, 28.3562) centre (33.7058, 28.3803) ccw
  arc A253 (53.9242, 52.8264) -> (53.5996, 53.1509) centre (53.5996, 52.8263) ccw
  line L58 (53.9242, 53.6829) -> (53.9242, 54.0724)
  line L59 (53.2751, 54.0724) -> (53.2751, 53.6829)
  arc A254 (29.8196, 28.6399) -> (29.7688, 28.6399) centre (29.7942, 28.6399) ccw
  line L60 (53.2751, 53.6829) -> (52.7558, 53.6829)
  line L61 (55.6204, 53.1509) -> (56.1396, 53.1509)
  line L62 (55.2958, 52.5018) -> (55.2958, 52.8264)
  arc A255 (56.1396, 53.1255) -> (56.1396, 53.1763) centre (56.1396, 53.1509) ccw
  arc A256 (61.5442, 52.8264) -> (61.2196, 53.1509) centre (61.2196, 52.8263) ccw
  arc A257 (56.23, 54.332) -> (56.1792, 54.332) centre (56.2046, 54.332) ccw
  arc A258 (58.1604, 53.1763) -> (58.1604, 53.1255) centre (58.1604, 53.1509) ccw
  line L63 (59.0042, 53.6829) -> (59.0042, 54.0075)
  arc A259 (59.0042, 54.0075) -> (58.3551, 54.0075) centre (58.6797, 54.0075) ccw
  arc A260 (55.3028, 53.967) -> (55.2888, 53.9181) centre (55.2958, 53.9426) ccw
  arc A261 (58.1604, 53.1509) -> (57.8358, 52.8264) centre (58.1604, 52.8263) ccw
  line L64 (56.2046, 53.6829) -> (56.2046, 54.332)
  arc A262 (58.3297, 54.0075) -> (58.3805, 54.0075) centre (58.3551, 54.0075) ccw
  arc A263 (57.8612, 52.8264) -> (57.8104, 52.8264) centre (57.8358, 52.8264) ccw
  arc A264 (57.8104, 53.6829) -> (57.8612, 53.6829) centre (57.8358, 53.6829) ccw
  arc A265 (56.1792, 53.6829) -> (56.23, 53.6829) centre (56.2046, 53.6829) ccw
  arc A266 (58.1604, 53.1255) -> (58.1604, 53.1763) centre (58.1604, 53.1509) ccw
  arc A267 (58.3551, 54.0724) -> (57.8358, 54.0724) centre (58.0954, 54.0724) ccw
  arc A268 (56.4896, 52.8264) -> (56.4388, 52.8264) centre (56.4642, 52.8264) ccw
  arc A269 (58.3297, 54.0724) -> (58.3805, 54.0724) centre (58.3551, 54.0724) ccw
  arc A270 (59.0296, 52.8264) -> (58.9788, 52.8264) centre (59.0042, 52.8264) ccw
  arc A271 (60.3758, 52.5272) -> (60.3758, 52.4764) centre (60.3758, 52.5018) ccw
  arc A272 (61.5442, 52.4764) -> (61.5442, 52.5272) centre (61.5442, 52.5018) ccw
  line L65 (61.5442, 52.5018) -> (60.3758, 52.5018)
  arc A273 (58.3297, 53.8127) -> (58.3805, 53.8127) centre (58.3551, 53.8127) ccw
  arc A274 (60.4012, 52.8264) -> (60.3504, 52.8264) centre (60.3758, 52.8264) ccw
  line L66 (59.0042, 52.5018) -> (57.8358, 52.5018)
  line L67 (55.9449, 54.1373) -> (56.4642, 54.1373)
  line L68 (59.0042, 52.8264) -> (59.0042, 52.5018)
  arc A275 (58.9788, 53.6829) -> (59.0296, 53.6829) centre (59.0042, 53.6829) ccw
  arc A276 (60.7004, 53.1509) -> (60.3758, 52.8264) centre (60.7004, 52.8263) ccw
  arc A277 (57.8104, 52.5018) -> (57.8612, 52.5018) centre (57.8358, 52.5018) ccw
  line L69 (60.7004, 53.1509) -> (61.2196, 53.1509)
  arc A278 (59.0042, 52.8264) -> (58.6796, 53.1509) centre (58.6796, 52.8263) ccw
  arc A279 (58.9788, 52.8264) -> (59.0296, 52.8264) centre (59.0042, 52.8264) ccw
  arc A280 (60.3504, 52.8264) -> (60.4012, 52.8264) centre (60.3758, 52.8264) ccw
  arc A281 (57.8612, 54.0724) -> (57.8104, 54.0724) centre (57.8358, 54.0724) ccw
  arc A282 (60.7004, 53.1763) -> (60.7004, 53.1255) centre (60.7004, 53.1509) ccw
  arc A283 (55.9449, 54.1627) -> (55.9449, 54.1119) centre (55.9449, 54.1373) ccw
  line L70 (57.8358, 52.5018) -> (57.8358, 52.8264)
  arc A284 (57.8104, 52.8264) -> (57.8612, 52.8264) centre (57.8358, 52.8264) ccw
  arc A285 (60.7004, 53.1255) -> (60.7004, 53.1763) centre (60.7004, 53.1509) ccw
  line L71 (58.3551, 54.0724) -> (58.3551, 53.8127)
  arc A286 (55.6204, 53.1763) -> (55.6204, 53.1255) centre (55.6204, 53.1509) ccw
  arc A287 (57.8358, 52.5272) -> (57.8358, 52.4764) centre (57.8358, 52.5018) ccw
  arc A288 (59.0042, 52.4764) -> (59.0042, 52.5272) centre (59.0042, 52.5018) ccw
  arc A289 (56.4642, 52.8264) -> (56.1396, 53.1509) centre (56.1396, 52.8263) ccw
  arc A290 (58.9788, 54.0075) -> (59.0296, 54.0075) centre (59.0042, 54.0075) ccw
  arc A291 (56.4388, 52.5018) -> (56.4896, 52.5018) centre (56.4642, 52.5018) ccw
  line L72 (56.4642, 52.8264) -> (56.4642, 52.5018)
  arc A292 (56.1976, 53.6585) -> (56.2115, 53.7073) centre (56.2045, 53.6829) ccw
  arc A293 (56.4642, 54.1119) -> (56.4642, 54.1627) centre (56.4642, 54.1373) ccw
  arc A294 (58.6796, 53.1255) -> (58.6796, 53.1763) centre (58.6796, 53.1509) ccw
  arc A295 (58.6796, 53.1763) -> (58.6796, 53.1255) centre (58.6796, 53.1509) ccw
  arc A296 (59.0296, 54.0075) -> (58.9788, 54.0075) centre (59.0042, 54.0075) ccw
  line L73 (58.1604, 53.1509) -> (58.6796, 53.1509)
  arc A297 (58.9788, 52.5018) -> (59.0296, 52.5018) centre (59.0042, 52.5018) ccw
  line L74 (55.2958, 53.9425) -> (56.2046, 53.6829)
  arc A298 (58.3805, 54.0724) -> (58.3297, 54.0724) centre (58.3551, 54.0724) ccw
  line L75 (57.8358, 53.6829) -> (57.8358, 54.0724)
  arc A299 (56.1396, 53.1763) -> (56.1396, 53.1255) centre (56.1396, 53.1509) ccw
  line L76 (60.3758, 52.5018) -> (60.3758, 52.8264)
  arc A300 (57.8104, 54.0724) -> (57.8612, 54.0724) centre (57.8358, 54.0724) ccw
  arc A301 (60.3504, 52.5018) -> (60.4012, 52.5018) centre (60.3758, 52.5018) ccw
  arc A302 (61.2196, 53.1255) -> (61.2196, 53.1763) centre (61.2196, 53.1509) ccw
  arc A303 (31.1578, 28.4044) -> (31.1738, 28.3562) centre (31.1658, 28.3803) ccw
  arc A304 (32.3422, 28.7456) -> (32.3262, 28.7938) centre (32.3342, 28.7697) ccw
  arc A305 (32.3262, 27.9667) -> (32.3422, 28.0149) centre (32.3342, 27.9908) ccw
  arc A306 (31.1738, 28.4044) -> (31.1578, 28.3562) centre (31.1658, 28.3803) ccw
  line L77 (31.4254, 29.1987) -> (31.1658, 29.5233)
  line L78 (61.5442, 53.6829) -> (61.5442, 54.332)
  line L79 (58.1604, 9.5899) -> (58.6796, 9.5899)
  arc A307 (60.6679, 54.3066) -> (60.6679, 54.3574) centre (60.6679, 54.332) ccw
  arc A308 (61.2196, 53.1763) -> (61.2196, 53.1255) centre (61.2196, 53.1509) ccw
  arc A309 (60.6276, 53.6587) -> (60.6433, 53.7071) centre (60.6355, 53.6829) ccw
  arc A310 (60.8951, 54.2346) -> (60.6679, 54.332) centre (60.6679, 54.0183) ccw
  line L80 (57.8358, 8.9408) -> (57.8358, 9.2654)
  arc A311 (61.5188, 52.5018) -> (61.5696, 52.5018) centre (61.5442, 52.5018) ccw
  arc A312 (60.6679, 54.332) -> (60.3758, 54.0399) centre (60.6679, 54.0399) ccw
  arc A313 (61.5696, 54.332) -> (61.5188, 54.332) centre (61.5442, 54.332) ccw
  line L81 (57.8358, 10.4465) -> (59.0042, 10.4465)
  line L82 (28.6258, 28.2504) -> (28.6258, 28.6399)
  arc A314 (57.8358, 8.9662) -> (57.8358, 8.9154) centre (57.8358, 8.9408) ccw
  line L83 (59.0042, 8.9408) -> (57.8358, 8.9408)
  arc A315 (57.8556, 10.4623) -> (57.816, 10.4306) centre (57.8358, 10.4465) ccw
  line L84 (59.0042, 10.1219) -> (59.0042, 10.771)
  arc A316 (32.3342, 29.4979) -> (32.3342, 29.5487) centre (32.3342, 29.5233) ccw
  arc A317 (60.4012, 54.0399) -> (60.3504, 54.0399) centre (60.3758, 54.0399) ccw
  arc A318 (60.6679, 54.3574) -> (60.6679, 54.3066) centre (60.6679, 54.332) ccw
  arc A319 (58.9788, 8.9408) -> (59.0296, 8.9408) centre (59.0042, 8.9408) ccw
  arc A320 (58.9788, 9.2654) -> (59.0296, 9.2654) centre (59.0042, 9.2654) ccw
  line L85 (61.5442, 52.8264) -> (61.5442, 52.5018)
  arc A321 (61.5696, 52.8264) -> (61.5188, 52.8264) centre (61.5442, 52.8264) ccw
  arc A322 (32.0167, 28.0882) -> (32.0675, 28.0882) centre (32.0421, 28.0882) ccw
  line L86 (32.3342, 29.1987) -> (32.3342, 29.8478)
  arc A323 (59.0042, 8.9154) -> (59.0042, 8.9662) centre (59.0042, 8.9408) ccw
  arc A324 (57.8358, 10.4718) -> (57.8358, 10.4211) centre (57.8358, 10.4465) ccw
  arc A325 (31.1658, 29.5487) -> (31.1658, 29.4979) centre (31.1658, 29.5233) ccw
  arc A326 (61.5188, 53.6829) -> (61.5696, 53.6829) centre (61.5442, 53.6829) ccw
  arc A327 (57.8612, 9.2654) -> (57.8104, 9.2654) centre (57.8358, 9.2654) ccw
  arc A328 (60.3758, 54.0399) -> (60.6354, 53.6829) centre (60.751, 54.0399) ccw
  arc A329 (61.5277, 53.6635) -> (61.5607, 53.7023) centre (61.5442, 53.6829) ccw
  line L87 (58.0954, 10.1219) -> (57.8358, 10.4465)
  arc A330 (59.0296, 9.2654) -> (58.9788, 9.2654) centre (59.0042, 9.2654) ccw
  arc A331 (58.1604, 9.5899) -> (57.8358, 9.2654) centre (58.1604, 9.2653) ccw
  arc A332 (60.3504, 54.0399) -> (60.4012, 54.0399) centre (60.3758, 54.0399) ccw
  arc A333 (58.6796, 9.5645) -> (58.6796, 9.6153) centre (58.6796, 9.5899) ccw
  arc A334 (59.0042, 10.4211) -> (59.0042, 10.4718) centre (59.0042, 10.4465) ccw
  arc A335 (61.5188, 52.8264) -> (61.5696, 52.8264) centre (61.5442, 52.8264) ccw
  arc A336 (60.9115, 54.254) -> (60.8786, 54.2153) centre (60.895, 54.2347) ccw
  line L88 (59.0042, 9.2654) -> (59.0042, 8.9408)
  arc A337 (31.4056, 29.1828) -> (31.4453, 29.2146) centre (31.4255, 29.1987) ccw
  arc A338 (31.1856, 29.5391) -> (31.146, 29.5074) centre (31.1658, 29.5233) ccw
  line L89 (34.8742, 27.9908) -> (33.7058, 28.3803)
  line L90 (31.1658, 29.5233) -> (32.3342, 29.5233)
  arc A339 (60.8767, 54.2171) -> (60.9135, 54.2522) centre (60.8951, 54.2346) ccw
  arc A340 (57.8104, 8.9408) -> (57.8612, 8.9408) centre (57.8358, 8.9408) ccw
  arc A341 (32.3088, 29.1987) -> (32.3596, 29.1987) centre (32.3342, 29.1987) ccw
  arc A342 (57.8104, 9.2654) -> (57.8612, 9.2654) centre (57.8358, 9.2654) ccw
  line L91 (34.5821, 28.6724) -> (34.5821, 28.0882)
  arc A343 (59.0042, 9.2654) -> (58.6796, 9.5899) centre (58.6796, 9.2653) ccw
  arc A344 (58.1604, 9.5645) -> (58.1604, 9.6153) centre (58.1604, 9.5899) ccw
  arc A345 (58.0756, 10.106) -> (58.1153, 10.1378) centre (58.0954, 10.1219) ccw
  line L92 (60.8951, 54.2346) -> (61.5442, 53.6829)
  arc A346 (32.3596, 29.8478) -> (32.3088, 29.8478) centre (32.3342, 29.8478) ccw
  arc A347 (58.6796, 9.6153) -> (58.6796, 9.5645) centre (58.6796, 9.5899) ccw
  line L93 (33.7058, 28.3803) -> (34.8742, 28.7697)
  arc A348 (58.1604, 9.6153) -> (58.1604, 9.5645) centre (58.1604, 9.5899) ccw
  arc A349 (32.0675, 28.6724) -> (32.0167, 28.6724) centre (32.0421, 28.6724) ccw
  arc A350 (28.6258, 29.2354) -> (28.6258, 29.1846) centre (28.6258, 29.21) ccw
  line L94 (70.485, 34.29) -> (52.07, 34.29)
  arc A351 (51.9938, 34.29) -> (52.1462, 34.29) centre (52.07, 34.29) ccw
  arc A352 (29.1705, 28.6399) -> (29.1197, 28.6399) centre (29.1451, 28.6399) ccw
  arc A353 (29.8065, 29.8369) -> (29.7819, 29.8813) centre (29.7942, 29.8591) ccw
  arc A354 (26.9946, 29.8986) -> (26.9946, 29.9494) centre (26.9946, 29.924) ccw
  arc A355 (29.7942, 52.6429) -> (29.7434, 52.6429) centre (29.7688, 52.6429) ccw
  arc A356 (29.7942, 30.4038) -> (29.7942, 30.4546) centre (29.7942, 30.4292) ccw
  arc A357 (29.7688, 52.2534) -> (30.0284, 51.9938) centre (30.0284, 52.2534) ccw
  arc A358 (28.9504, 31.0783) -> (28.6258, 30.7537) centre (28.9504, 30.7537) ccw
  line L95 (26.0858, 29.2749) -> (26.0858, 29.924)
  arc A359 (52.07, 40.7162) -> (52.07, 40.5638) centre (52.07, 40.64) ccw
  arc A360 (70.4088, 34.29) -> (70.5612, 34.29) centre (70.485, 34.29) ccw
  arc A361 (52.1462, 40.64) -> (51.9938, 40.64) centre (52.07, 40.64) ccw
  arc A362 (29.7942, 30.7537) -> (29.4696, 31.0783) centre (29.4696, 30.7537) ccw
  arc A363 (28.6004, 30.7537) -> (28.6512, 30.7537) centre (28.6258, 30.7537) ccw
  arc A364 (28.9504, 31.0529) -> (28.9504, 31.1037) centre (28.9504, 31.0783) ccw
  line L96 (31.1658, 28.3803) -> (32.3342, 28.7697)
  arc A365 (28.6512, 28.2504) -> (28.6004, 28.2504) centre (28.6258, 28.2504) ccw
  arc A366 (70.485, 40.5638) -> (70.485, 40.7162) centre (70.485, 40.64) ccw
  line L97 (29.7688, 52.2534) -> (29.7688, 52.6429)
  arc A367 (29.7942, 52.2534) -> (29.7434, 52.2534) centre (29.7688, 52.2534) ccw
  arc A368 (28.6135, 29.2322) -> (28.6381, 29.1878) centre (28.6258, 29.21) ccw
  arc A369 (28.6258, 30.4546) -> (28.6258, 30.4038) centre (28.6258, 30.4292) ccw
  line L98 (28.6258, 30.4292) -> (28.6258, 30.7537)
  arc A370 (28.9504, 31.1037) -> (28.9504, 31.0529) centre (28.9504, 31.0783) ccw
  arc A371 (70.485, 34.2138) -> (70.485, 34.3662) centre (70.485, 34.29) ccw
  line L99 (29.7688, 53.213) -> (30.9372, 53.8621)
  arc A372 (50.9947, 29.9494) -> (50.9947, 29.8986) centre (50.9947, 29.924) ccw
  arc A373 (28.6512, 30.7537) -> (28.6004, 30.7537) centre (28.6258, 30.7537) ccw
  arc A374 (29.4696, 31.1037) -> (29.4696, 31.0529) centre (29.4696, 31.0783) ccw
  arc A375 (29.7688, 53.2384) -> (29.7688, 53.1876) centre (29.7688, 53.213) ccw
  arc A376 (52.07, 34.3662) -> (52.07, 34.2138) centre (52.07, 34.29) ccw
  arc A377 (29.7688, 30.4292) -> (29.8196, 30.4292) centre (29.7942, 30.4292) ccw
  arc A378 (29.8196, 30.7537) -> (29.7688, 30.7537) centre (29.7942, 30.7537) ccw
  line L100 (52.07, 40.64) -> (70.485, 40.64)
  line L101 (33.6042, 52.5018) -> (32.4358, 52.5018)
  arc A379 (28.8854, 27.9654) -> (28.8854, 28.0162) centre (28.8854, 27.9908) ccw
  arc A380 (28.6004, 30.4292) -> (28.6512, 30.4292) centre (28.6258, 30.4292) ccw
  line L102 (29.7942, 30.4292) -> (28.6258, 30.4292)
  arc A381 (29.7688, 30.7537) -> (29.8196, 30.7537) centre (29.7942, 30.7537) ccw
  line L103 (32.3342, 27.9908) -> (31.1658, 28.3803)
  arc A382 (29.5346, 27.9654) -> (29.5346, 28.0162) centre (29.5346, 27.9908) ccw
  line L104 (52.07, 34.29) -> (52.07, 40.64)
  line L105 (32.0421, 28.6724) -> (32.0421, 28.0882)
  arc A383 (30.0284, 51.9684) -> (30.0284, 52.0192) centre (30.0284, 51.9938) ccw
  arc A384 (28.6258, 29.8845) -> (28.6258, 29.8337) centre (28.6258, 29.8591) ccw
  arc A385 (29.7434, 52.2534) -> (29.7942, 52.2534) centre (29.7688, 52.2534) ccw
  arc A386 (29.7942, 29.8337) -> (29.7942, 29.8845) centre (29.7942, 29.8591) ccw
  arc A387 (54.6885, 2.5146) -> (54.6885, 2.4638) centre (54.6885, 2.4892) ccw
  arc A388 (54.9481, 1.2954) -> (54.9481, 1.3462) centre (54.9481, 1.3208) ccw
  arc A389 (51.1246, 29.9494) -> (51.1246, 29.8986) centre (51.1246, 29.924) ccw
  line L106 (70.485, 40.64) -> (70.485, 34.29)
  arc A390 (29.7942, 29.1846) -> (29.7942, 29.2354) centre (29.7942, 29.21) ccw
  arc A391 (28.6258, 28.2504) -> (28.8854, 27.9908) centre (28.8854, 28.2504) ccw
  arc A392 (70.5612, 40.64) -> (70.4088, 40.64) centre (70.485, 40.64) ccw
  arc A393 (28.6004, 28.2504) -> (28.6512, 28.2504) centre (28.6258, 28.2504) ccw
  line L107 (29.7942, 30.7537) -> (29.7942, 30.4292)